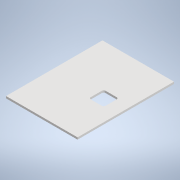
# Autodesk Inventor part: plate2
Saved by Autodesk Inventor 2020 (Build 240168000, 168)
## iProperties
Created: 2020-07-26
Part Number: plate2
Material: Stainless Steel
Document SubType Name: Modeling
Designer: Aarya
Density: 8 g/cm^3
Appearance: Semi-Polished
Author: Aarya
Autodesk Inventor part; units mm, degrees
ref_plane "YZ Plane" through (0, 0, 0) normal (1, 0, 0) x (0, 1, 0)
ref_plane "XZ Plane" through (0, 0, 0) normal (0, 1, 0) x (-1, 0, 0)
ref_plane "XY Plane" through (0, 0, 0) normal (0, 0, 1) x (1, 0, 0)
sketch "Sketch1" plane through (0, 0, 0) normal (0, 1, 0) x (-1, 0, 0)
  line L0 (31, 48.6655) -> (-31, 48.6655)
  line L1 (-31, 48.6655) -> (-31, -48.6655)
  line L2 (-31, -48.6655) -> (31, -48.6655)
  line L3 (31, -48.6655) -> (31, 48.6655)
  line L4 (31, 48.6655) -> (-31, -48.6655) construction
  line L5 (-31, 48.6655) -> (31, -48.6655) construction
  point P0 (0, 0)
  dimension "d0" = 97.331
  dimension "d1" = 62
  constraints: 12 end point, 2 midpoint, 2 parallel, 1 horizontal, 1 perpendicular
  measures "d0" distance of L2.end L0.start
  measures "d1" distance of L0.start L0.end
extrude "Extrusion1" add sketch "Sketch1" along normal blind 2
sketch "Sketch2" plane through (0, 2, 0) normal (0, 1, 0) x (1, 0, 0)
  line L0 (9.6595, -8.8304) -> (20.6595, -8.8304) projected
  arc A0 (20.6595, -8.8304) -> (22.6595, -6.8304) centre (20.6595, -6.8304) ccw projected
  line L1 (22.6595, -6.8304) -> (22.6595, 4.1696) projected
  arc A1 (22.6595, 4.1696) -> (20.6595, 6.1696) centre (20.6595, 4.1696) ccw projected
  line L2 (20.6595, 6.1696) -> (9.6595, 6.1696) projected
  arc A2 (9.6595, 6.1696) -> (7.6595, 4.1696) centre (9.6595, 4.1696) ccw projected
  line L3 (7.6595, 4.1696) -> (7.6595, -6.8304) projected
  arc A3 (7.6595, -6.8304) -> (9.6595, -8.8304) centre (9.6595, -6.8304) ccw projected
  line L4 (14.1595, 0.1696) -> (9.6595, 0.1696) projected
  line L5 (9.6595, 0.1696) -> (9.6595, 3.1696) projected
  line L6 (9.6595, 3.1696) -> (14.1595, 3.1696) projected
  line L7 (14.1595, 3.1696) -> (14.1595, 0.1696) projected
  line L8 (16.1595, -5.8304) -> (16.1595, -2.8304) projected
  line L9 (16.1595, -2.8304) -> (20.6595, -2.8304) projected
  line L10 (20.6595, -2.8304) -> (20.6595, -5.8304) projected
  line L11 (20.6595, -5.8304) -> (16.1595, -5.8304) projected
  line L12 (16.1595, 3.1696) -> (20.6595, 3.1696) projected
  line L13 (20.6595, 3.1696) -> (20.6595, 0.1696) projected
  line L14 (20.6595, 0.1696) -> (16.1595, 0.1696) projected
  line L15 (16.1595, 0.1696) -> (16.1595, 3.1696) projected
  line L16 (9.6595, -2.8304) -> (14.1595, -2.8304) projected
  line L17 (14.1595, -2.8304) -> (14.1595, -5.8304) projected
  line L18 (14.1595, -5.8304) -> (9.6595, -5.8304) projected
  line L19 (9.6595, -5.8304) -> (9.6595, -2.8304) projected
  point P0 (0, 0)
extrude "Extrusion2" cut sketch "Sketch2" against normal blind 10 contours A3 L3 A2 L2 A1 L1 A0 L0 | L4 L5 L6 L7 | L8 L9 L10 L11 | L12 L13 L14 L15 | L16 L17 L18 L19
body "Solid1"
